006 (Autodesk Fusion 360 design; units mm, degrees)
Autodesk Fusion 360 part; units mm, degrees
sketch "Esquisse1" plane through (0, 0, 0) normal (1, 0, 0) x (0, 1, 0)
  line L0 (-50, 85) -> (50, 85)
  line L1 (50, 85) -> (50, 0)
  line L2 (50, 0) -> (-50, 0)
  line L3 (-50, 0) -> (-50, 85)
  line L4 (0, 1.75) -> (0, 22.5)
  dimension "d1" = 85
  dimension "d2" = 100
  constraint horizontal L0
  constraint vertical L1
  constraint horizontal L2
  constraint vertical L3
  constraint coincident origin L2
  constraint symmetric L1 L3 L4
  measures "d1" distance of L0.start L2.end
  measures "d2" distance of L0.start L0.end
extrude "Extrusion1" add sketch "Esquisse1" along normal blind 30
sketch "Esquisse2" plane through (0, 0, 0) normal (-1, 0, 0) x (0, -1, 0)
  line L0 (-50, 0) -> (50, 0)
  line L1 (50, 0) -> (50, 85)
  line L2 (50, 85) -> (-50, 85)
  line L3 (-50, 85) -> (-50, 0)
  circle A0 centre (-35, 72.5) radius 4.075
  line L4 (0, 1.75) -> (0, 22.5)
  dimension "d5" = 8.15
  dimension "d6" = 12.5
  dimension "d7" = 35
  measures "d5" diameter of A0
  measures "d6" distance of L2 A0.centre
  measures "d7" distance of A0.centre L4
extrude "Extrusion2" cut sketch "Esquisse2" against normal blind 40 contours A0
mirror "Symétrie miroir1" about plane through (0, 0, 0) normal (0, 1, 0) of "Extrusion2"
equation "d7 = ( 70 / 2 ) * 1 mm"
